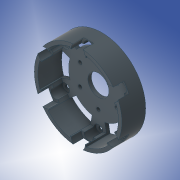
# Autodesk Inventor part: SJ002
Saved by Autodesk Inventor 2017 SP1 (Build 210196100, 196)
## iProperties
Created: 2017-06-01
Part Number: SJ002
Material: ABS Plastic
Document SubType Name: Modeling
Designer: Zach
Density: 1.06 g/cm^3
Appearance: CR Dark Blue
Mass: 108.284 g
Surface Area: 474.294 cm^2
Volume: 102.155 cm^3
Author: Zach
Autodesk Inventor part; units mm, degrees
ref_plane "YZ Plane" through (0, 0, 0) normal (1, 0, 0) x (0, 1, 0)
ref_plane "XZ Plane" through (0, 0, 0) normal (0, 1, 0) x (-1, 0, 0)
ref_plane "XY Plane" through (0, 0, 0) normal (0, 0, 1) x (1, 0, 0)
sketch "Sketch2" plane through (0, 0, 0) normal (0, 0, 1) x (1, 0, 0)
  circle A0 centre (0, 0) radius 62.5
  circle A1 centre (0, 0) radius 15
  dimension "d0" = 125
  dimension "d1" = 30
  constraints: 2 centre point, 2 coincident
  measures "d0" diameter of A0
  measures "d1" diameter of A1
extrude "Extrusion1" add sketch "Sketch2" along normal blind 10
sketch "Sketch4" plane through (0, 0, 0) normal (0, 0, -1) x (-1, 0, 0)
  circle A0 centre (0, 30) radius 2.575
  circle A1 centre (-25.9808, 15) radius 2.575
  circle A2 centre (-25.9808, -15) radius 2.575
  circle A3 centre (0, -30) radius 2.575
  circle A4 centre (25.9808, -15) radius 2.575
  circle A5 centre (25.9808, 15) radius 2.575
  point P0 (0, 0)
  dimension "d8" = 5.15
  dimension "d9" = 30
  dimension "d12" = 360
  constraints: 6 centre point, 1 vertical alignment, 13 other
  measures "d8" diameter of A0
  measures "d9" distance of point (0, 0) A0.centre
extrude "Extrusion3" cut sketch "Sketch4" against normal through all
sketch "Sketch5" plane through (0, 0, 10) normal (0, 0, 1) x (1, 0, 0)
  circle A0 centre (0, 0) radius 55
  dimension "d16" = 110
  constraints: 1 centre point, 1 coincident
  measures "d16" diameter of A0
extrude "Extrusion4" cut sketch "Sketch5" against normal blind 5
sketch "Sketch6" plane through (0, 0, 10) normal (0, 0, 1) x (1, 0, 0)
  circle A0 centre (0, 55) radius 2.5
  circle A1 centre (-47.6314, 27.5) radius 2.5
  circle A2 centre (-47.6314, -27.5) radius 2.5
  circle A3 centre (0, -55) radius 2.5
  circle A4 centre (47.6314, -27.5) radius 2.5
  circle A5 centre (47.6314, 27.5) radius 2.5
  point P0 (0, 0)
  dimension "d19" = 5
  dimension "d20" = 55
  dimension "d23" = 360
  constraints: 6 centre point, 13 other
  measures "d19" diameter of A0
  measures "d20" distance of point (0, 0) A0.centre
extrude "Extrusion5" cut sketch "Sketch6" against normal through all
sketch "Sketch8" plane through (0, 0, 10) normal (0, 0, 1) x (1, 0, 0)
  arc A0 (48.8319, -25.3071) -> (48.8319, 25.3071) centre (0, 0) ccw projected
  circle A1 centre (0, 0) radius 62.5 projected
  circle A2 centre (0, 55) radius 2.5 projected
  circle A3 centre (0, 55) radius 6.5
  circle A4 centre (-47.6314, 27.5) radius 6.5
  circle A5 centre (-47.6314, -27.5) radius 6.5
  circle A6 centre (0, -55) radius 6.5
  circle A7 centre (47.6314, -27.5) radius 6.5
  circle A8 centre (47.6314, 27.5) radius 6.5
  arc A9 (46.3325, -29.6361) -> (48.8319, -25.3071) centre (47.6314, -27.5) ccw projected
  arc A10 (2.4994, -54.9432) -> (46.3325, -29.6361) centre (0, 0) ccw projected
  arc A11 (-2.4994, -54.9432) -> (2.4994, -54.9432) centre (0, -55) ccw projected
  arc A12 (-46.3325, -29.6361) -> (-2.4994, -54.9432) centre (0, 0) ccw projected
  arc A13 (-48.8319, -25.3071) -> (-46.3325, -29.6361) centre (-47.6314, -27.5) ccw projected
  arc A14 (-48.8319, 25.3071) -> (-48.8319, -25.3071) centre (0, 0) ccw projected
  arc A15 (-46.3325, 29.6361) -> (-48.8319, 25.3071) centre (-47.6314, 27.5) ccw projected
  arc A16 (-2.4994, 54.9432) -> (-46.3325, 29.6361) centre (0, 0) ccw projected
  arc A17 (2.4994, 54.9432) -> (-2.4994, 54.9432) centre (0, 55) ccw projected
  arc A18 (46.3325, 29.6361) -> (2.4994, 54.9432) centre (0, 0) ccw projected
  arc A19 (48.8319, 25.3071) -> (46.3325, 29.6361) centre (47.6314, 27.5) ccw projected
  point P0 (-56.2917, 32.5)
  point P1 (-56.2917, -32.5)
  point P2 (0, -65)
  point P3 (56.2917, -32.5)
  point P4 (56.2917, 32.5)
  dimension "d28" = 13
  dimension "d31" = 360
  constraints: 6 centre point, 1 coincident, 17 other
  measures "d28" diameter of A3
extrude "Extrusion6" cut sketch "Sketch8" against normal blind 5 contours A9 A10 A7 A0 | A0 A7 A10 A9 | A8 A18 A19 A0 | A0 A19 A18 A8 | A10 A11 A12 A6 | A6 A12 A11 A10 | A18 A2 A16 A3 | A3 A16 A2 A18 | A2 | A12 A13 A14 A5 | A5 A14 A13 A12 | A16 A15 A14 A4 | A4 A14 A15 A16
sketch "Sketch9" plane through (0, 0, 10) normal (0, 0, 1) x (1, 0, 0)
  circle A0 centre (0, 0) radius 15 construction
  circle A1 centre (0, 0) radius 42.5 construction
  circle A2 centre (0, 0) radius 57.5 construction
  line L0 (40.4629, 13) -> (54.61, 18)
  line L1 (40.4629, -13) -> (54.61, -18)
  line L2 (0, 0) -> (92.9665, 0) construction
  arc A3 (40.4629, -13) -> (40.4629, 13) centre (0, 0) ccw
  arc A4 (54.61, -18) -> (54.61, 18) centre (0, 0) ccw
  circle A5 centre (0, 0) radius 42.5 construction
  line L3 (8.9731, 41.5419) -> (11.7165, 56.2936)
  arc A6 (31.4898, 28.5419) -> (8.9731, 41.5419) centre (0, 0) ccw
  line L4 (31.4898, 28.5419) -> (42.8934, 38.2936)
  circle A7 centre (0, 0) radius 57.5 construction
  arc A8 (42.8934, 38.2936) -> (11.7165, 56.2936) centre (0, 0) ccw
  circle A9 centre (0, 0) radius 42.5 construction
  line L5 (-31.4898, 28.5419) -> (-42.8934, 38.2936)
  arc A10 (-8.9731, 41.5419) -> (-31.4898, 28.5419) centre (0, 0) ccw
  line L6 (-8.9731, 41.5419) -> (-11.7165, 56.2936)
  circle A11 centre (0, 0) radius 57.5 construction
  arc A12 (-11.7165, 56.2936) -> (-42.8934, 38.2936) centre (0, 0) ccw
  circle A13 centre (0, 0) radius 42.5 construction
  line L7 (-40.4629, -13) -> (-54.61, -18)
  arc A14 (-40.4629, 13) -> (-40.4629, -13) centre (0, 0) ccw
  line L8 (-40.4629, 13) -> (-54.61, 18)
  circle A15 centre (0, 0) radius 57.5 construction
  arc A16 (-54.61, 18) -> (-54.61, -18) centre (0, 0) ccw
  circle A17 centre (0, 0) radius 42.5 construction
  line L9 (-8.9731, -41.5419) -> (-11.7165, -56.2936)
  arc A18 (-31.4898, -28.5419) -> (-8.9731, -41.5419) centre (0, 0) ccw
  line L10 (-31.4898, -28.5419) -> (-42.8934, -38.2936)
  circle A19 centre (0, 0) radius 57.5 construction
  arc A20 (-42.8934, -38.2936) -> (-11.7165, -56.2936) centre (0, 0) ccw
  circle A21 centre (0, 0) radius 42.5 construction
  line L11 (31.4898, -28.5419) -> (42.8934, -38.2936)
  arc A22 (8.9731, -41.5419) -> (31.4898, -28.5419) centre (0, 0) ccw
  line L12 (8.9731, -41.5419) -> (11.7165, -56.2936)
  circle A23 centre (0, 0) radius 57.5 construction
  arc A24 (11.7165, -56.2936) -> (42.8934, -38.2936) centre (0, 0) ccw
  dimension "d35" = 85
  dimension "d36" = 115
  dimension "d37" = 13
  dimension "d38" = 18
  dimension "d41" = 360
  constraints: 48 point on circle, 26 end point, 24 centre point, 12 concentric, 7 coincident, 1 horizontal, 86 other
  measures "d35" diameter of A1
  measures "d36" diameter of A2
  measures "d37" vertical distance of L0.start point (0, 0)
  measures "d38" vertical distance of L0.end point (0, 0)
extrude "Extrusion7" cut sketch "Sketch9" against normal through all
sketch "Sketch11" plane through (0, 0, 10) normal (0, 0, 1) x (1, 0, 0)
  line L0 (-42.8934, -38.2936) -> (-40.993, -36.6685) projected
  arc A0 (-44.0544, -32.9273) -> (-40.993, -36.6685) centre (0, 0) ccw projected
  arc A1 (-50.5431, -21.6886) -> (-44.0544, -32.9273) centre (-47.6314, -27.5) ccw projected
  arc A2 (-52.2523, -17.1667) -> (-50.5431, -21.6886) centre (0, 0) ccw projected
  line L1 (-52.2523, -17.1667) -> (-54.61, -18) projected
  arc A3 (-54.61, 18) -> (-54.61, -18) centre (0, 0) ccw projected
  line L2 (-54.61, 18) -> (-52.2523, 17.1667) projected
  arc A4 (-50.5431, 21.6886) -> (-52.2523, 17.1667) centre (0, 0) ccw projected
  arc A5 (-44.0544, 32.9273) -> (-50.5431, 21.6886) centre (-47.6314, 27.5) ccw projected
  arc A6 (-40.993, 36.6685) -> (-44.0544, 32.9273) centre (0, 0) ccw projected
  line L3 (-40.993, 36.6685) -> (-42.8934, 38.2936) projected
  arc A7 (-11.7165, 56.2936) -> (-42.8934, 38.2936) centre (0, 0) ccw projected
  line L4 (-11.7165, 56.2936) -> (-11.2593, 53.8352) projected
  arc A8 (-6.4886, 54.6159) -> (-11.2593, 53.8352) centre (0, 0) ccw projected
  arc A9 (6.4886, 54.6159) -> (-6.4886, 54.6159) centre (0, 55) ccw projected
  arc A10 (11.2593, 53.8352) -> (6.4886, 54.6159) centre (0, 0) ccw projected
  line L5 (11.2593, 53.8352) -> (11.7165, 56.2936) projected
  arc A11 (42.8934, 38.2936) -> (11.7165, 56.2936) centre (0, 0) ccw projected
  line L6 (42.8934, 38.2936) -> (40.993, 36.6685) projected
  arc A12 (44.0544, 32.9273) -> (40.993, 36.6685) centre (0, 0) ccw projected
  arc A13 (50.5431, 21.6886) -> (44.0544, 32.9273) centre (47.6314, 27.5) ccw projected
  arc A14 (52.2523, 17.1667) -> (50.5431, 21.6886) centre (0, 0) ccw projected
  line L7 (52.2523, 17.1667) -> (54.61, 18) projected
  arc A15 (54.61, -18) -> (54.61, 18) centre (0, 0) ccw projected
  line L8 (54.61, -18) -> (52.2523, -17.1667) projected
  arc A16 (50.5431, -21.6886) -> (52.2523, -17.1667) centre (0, 0) ccw projected
  arc A17 (44.0544, -32.9273) -> (50.5431, -21.6886) centre (47.6314, -27.5) ccw projected
  arc A18 (40.993, -36.6685) -> (44.0544, -32.9273) centre (0, 0) ccw projected
  line L9 (40.993, -36.6685) -> (42.8934, -38.2936) projected
  arc A19 (11.7165, -56.2936) -> (42.8934, -38.2936) centre (0, 0) ccw projected
  line L10 (11.7165, -56.2936) -> (11.2593, -53.8352) projected
  arc A20 (6.4886, -54.6159) -> (11.2593, -53.8352) centre (0, 0) ccw projected
  arc A21 (-6.4886, -54.6159) -> (6.4886, -54.6159) centre (0, -55) ccw projected
  arc A22 (-11.2593, -53.8352) -> (-6.4886, -54.6159) centre (0, 0) ccw projected
  line L11 (-11.2593, -53.8352) -> (-11.7165, -56.2936) projected
  arc A23 (-42.8934, -38.2936) -> (-11.7165, -56.2936) centre (0, 0) ccw projected
  circle A24 centre (0, 0) radius 62.5 projected
extrude "Extrusion8" add sketch "Sketch11" along normal blind 24
sketch "Sketch12" plane through (0, 0, 5) normal (0, 0, 1) x (1, 0, 0)
  circle A0 centre (47.6314, 27.5) radius 2.5 construction
  circle A1 centre (47.6314, 27.5) radius 6.5
  arc A2 (50.5431, 21.6886) -> (44.0544, 32.9273) centre (47.6314, 27.5) ccw projected
  circle A3 centre (47.6314, -27.5) radius 6.5
  circle A4 centre (0, -55) radius 6.5
  circle A5 centre (-47.6314, -27.5) radius 6.5
  circle A6 centre (-47.6314, 27.5) radius 6.5
  circle A7 centre (0, 55) radius 6.5
  point P0 (0, 0)
  dimension "d49" = 360
  constraints: 6 centre point, 2 concentric, 1 coincident, 13 other
extrude "Extrusion9" cut sketch "Sketch12" against normal blind 3
sketch "Sketch13" plane through (0, 0, 34) normal (0, 0, 1) x (1, 0, 0)
  circle A0 centre (47.6314, 27.5) radius 2.5 construction
  circle A1 centre (47.6314, 27.5) radius 6.5 construction
  circle A2 centre (47.6314, 27.5) radius 2.5 projected
  circle A3 centre (47.6314, 27.5) radius 10
  circle A4 centre (0, 55) radius 10
  circle A5 centre (-47.6314, 27.5) radius 10
  circle A6 centre (-47.6314, -27.5) radius 10
  circle A7 centre (0, -55) radius 10
  circle A8 centre (47.6314, -27.5) radius 10
  point P0 (0, 0)
  dimension "d53" = 20
  dimension "d56" = 360
  constraints: 6 centre point, 1 coincident, 13 other
  measures "d53" diameter of A3
extrude "Extrusion10" cut sketch "Sketch13" against normal blind 15 contours A2 | A3 | A4 | A5 | A6 | A7 | A8
body "Solid1"
